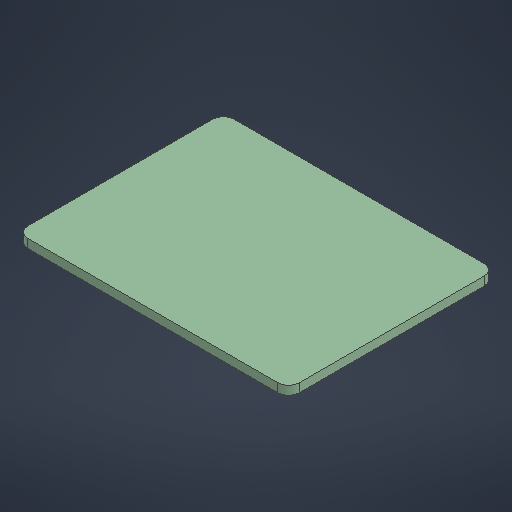
# Autodesk Inventor part: PCB
Saved by Autodesk Inventor 2026.1 (Build 301233020, 233B)
## iProperties
Created: 2026-05-23
Part Number: PCB
Material: Generic
Document SubType Name: Modeling
Designer: InventorKid
Density: 1 g/cm^3
Appearance: Default
Author: InventorKid
Autodesk Inventor part; units mm, degrees
ref_plane "YZ Plane" through (0, 0, 0) normal (1, 0, 0) x (0, 1, 0)
ref_plane "XZ Plane" through (0, 0, 0) normal (0, 1, 0) x (-1, 0, 0)
ref_plane "XY Plane" through (0, 0, 0) normal (0, 0, 1) x (1, 0, 0)
sketch "Sketch1" plane through (0, 0, 0) normal (0, 1, 0) x (-1, 0, 0)
  line L0 (0, 0) -> (50, 0)
  line L1 (50, 0) -> (50, -38)
  line L2 (50, -38) -> (0, -38)
  line L3 (0, -38) -> (0, 0)
  dimension "d0" = 38
  dimension "d1" = 50
  constraints: 8 end point, 2 parallel, 1 horizontal, 1 perpendicular
  measures "d0" distance of L2.end L0.start
  measures "d1" distance of L0.start L0.end
extrude "Extrusion1" add sketch "Sketch1" along normal blind 1.6
fillet "Fillet1" radius 2 4 edges at (0, 0.8, 0) (0, 0.8, -38) (-50, 0.8, -38) (-50, 0.8, 0)
body "Solid1"
